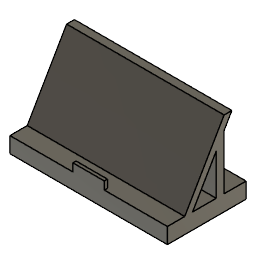
phone holder_ (Autodesk Fusion 360 design; units mm, degrees)
Autodesk Fusion 360 part; units mm, degrees
sketch "Sketch1" plane through (0, 0, 0) normal (0, 0, 1) x (1, 0, 0)
  line L0 (0, 0) -> (0, 50)
  line L1 (0, 50) -> (100, 50)
  line L2 (100, 50) -> (100, 0)
  line L3 (100, 0) -> (0, 0)
  dimension "d2" = 50
  dimension "d3" = 100
  dimension "d4" = 50
  constraint coincident L0.start L3.end
  constraint vertical L0
  constraint perpendicular L0 L1
  constraint perpendicular L1 L2
  measures "d2" distance of L0.start L0.end
  measures "d3" distance of L0.end L1.end
  measures "d4" distance of L1.end L2.end
extrude "Extrude1" add sketch "Sketch1" along normal blind 10
sketch "Sketch2" plane through (0, 0, 0) normal (1, 0, 0) x (0, 1, 0)
  line L0 (0, 10) -> (11, 10)
  line L1 (11, 10) -> (36, 53.3013) construction
  line L2 (11, 10) -> (36, 53.3013)
  line L3 (36, 53.3013) -> (41, 53.3013)
  line L4 (41, 53.3013) -> (16, 10)
  line L5 (16, 10) -> (11, 10)
  line L6 (41, 53.3013) -> (36, 44.641)
  line L7 (36, 44.641) -> (36, 10)
  line L8 (36, 10) -> (31, 10)
  line L9 (31, 10) -> (31, 35.9808)
  dimension "d7" = 11
  dimension "d10" = 50
  dimension "d11" = 5
  dimension "d12" = 10
  dimension "d13" = 5
  constraint horizontal L0
  constraint coincident L0.end L1.start
  constraint coincident L4 L6.end
  constraint perpendicular L3 L7
  constraint perpendicular L7 L8
  constraint coincident L4 L9.end
  constraint perpendicular L8 L9
  measures "d7" distance of L0.start L0.end
  measures "d10" distance of L1.end L0.end
  measures "d11" distance of L1.end L3.end
  measures "d12" distance of L3.end L6.end
  measures "d13" distance of L7.end L8.end
extrude "Extrude2" add sketch "Sketch2" along normal blind 100
sketch "Sketch3" plane through (0, 0, 10) normal (0, 0, 1) x (-1, 0, 0)
  line L0 (-100, -11) -> (0, -11)
  line L1 (0, -11) -> (0, 0)
  line L2 (0, 0) -> (-100, 0)
  line L3 (-100, 0) -> (-100, -11)
  line L4 (-50, 0) -> (-60, 0)
  line L5 (-50, 0) -> (-40, 0)
  line L6 (-60, 0) -> (-60, -2)
  line L7 (-60, -2) -> (-40, -2)
  line L8 (-40, -2) -> (-40, 0)
  dimension "d16" = 10
  dimension "d17" = 10
  dimension "d18" = 2
  constraint midpoint L2 L4.start
  constraint coincident L2 L4.end
  constraint coincident L2 L5.end
  constraint perpendicular L4 L6
  constraint perpendicular L6 L7
  constraint perpendicular L5 L8
  measures "d16" distance of L4.start L4.end
  measures "d17" distance of L4.start L5.end
  measures "d18" distance of L4.end L6.end
extrude "Extrude3" add sketch "Sketch3" along normal blind 5 contours L2 L4 L5 L6 L7 L8
